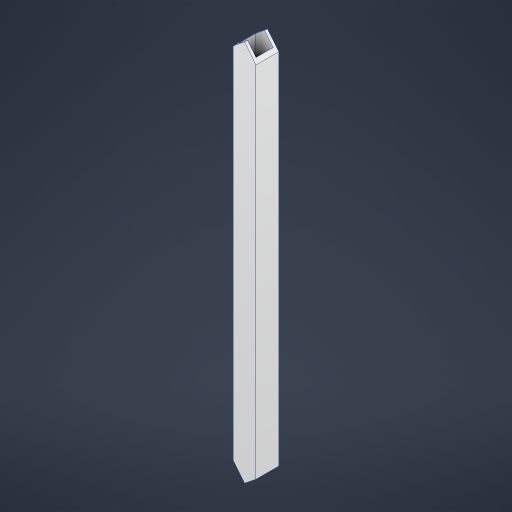
# Autodesk Inventor part: STRU_013_BilletCrossbar2_Angled
Saved by Autodesk Inventor 2024.2 (Build 282272000, 272)
## iProperties
Created: 2024-07-25
Part Number: STRU_013_BilletCrossbar2_Angled
Material: Aluminum 6061
Document SubType Name: Modeling
Designer: Bryan
Density: 2.7 g/cm^3
Appearance: Aluminum - Flat
Author: Bryan
Autodesk Inventor part; units mm, degrees
ref_plane "YZ Plane" through (0, 0, 0) normal (1, 0, 0) x (0, 1, 0)
ref_plane "XZ Plane" through (0, 0, 0) normal (0, 1, 0) x (-1, 0, 0)
ref_plane "XY Plane" through (0, 0, 0) normal (0, 0, 1) x (1, 0, 0)
sketch "Sketch1" plane through (0, 0, 0) normal (0, 1, 0) x (-1, 0, 0)
  line L0 (-12.7, -12.7) -> (12.7, -12.7)
  line L1 (12.7, -12.7) -> (12.7, 12.7)
  line L2 (12.7, 12.7) -> (-12.7, 12.7)
  line L3 (-12.7, 12.7) -> (-12.7, -12.7)
  line L4 (-12.7, -12.7) -> (12.7, 12.7) construction
  line L5 (12.7, -12.7) -> (-12.7, 12.7) construction
  line L6 (9.525, 9.525) -> (9.525, -9.525)
  line L7 (9.525, -9.525) -> (-9.525, -9.525)
  line L8 (-9.525, -9.525) -> (-9.525, 9.525)
  line L9 (-9.525, 9.525) -> (9.525, 9.525)
  point P0 (0, 0)
  dimension "d0" = 25.4
  dimension "d1" = 25.4
  dimension "d2" = 3.175
  constraints: 20 end point, 4 parallel, 2 midpoint, 2 perpendicular, 1 horizontal, 3 other
  measures "d0" distance of L2.end L1.end
  measures "d1" distance of L1.end L0.end
  measures "d2" distance between parallel lines of L1 L6
extrude "Extrusion1" add sketch "Sketch1" along normal blind 425.45
sketch "Sketch4" plane through (-12.7, 0, 12.7) normal (0, 0, 1) x (1, 0, 0)
  line L0 (220.4933, 167.1851) -> (12.7, 425.45)
  line L1 (12.7, 425.45) -> (-195.0933, 258.2649)
  line L2 (-195.0933, 258.2649) -> (12.7, 0)
  line L3 (12.7, 0) -> (220.4933, 167.1851)
  line L4 (0, 0) -> (25.4, 0) projected
  line L5 (0, 425.45) -> (25.4, 425.45) projected
  line L6 (0, 0) -> (25.4, 0) projected
  line L7 (25.4, 0) -> (25.4, 425.45) projected
  line L8 (0, 425.45) -> (25.4, 425.45) projected
  line L9 (0, 0) -> (0, 425.45) projected
  point P0 (0, 15.7847)
  point P1 (25.4, 10.2181)
  point P2 (0, 415.2319)
  point P3 (25.4, 409.6653)
  dimension "d13" = 266.7
  constraints: 8 end point, 2 midpoint, 2 parallel, 1 perpendicular
  measures "d13" distance of L0.end L1.end
extrude "Extrusion4" cut sketch "Sketch4" against normal blind 370.4968 contours L0 L5 L7 | L7 L4 L3 | L1 L9 L5 | L4 L9 L2
body "Solid1"
